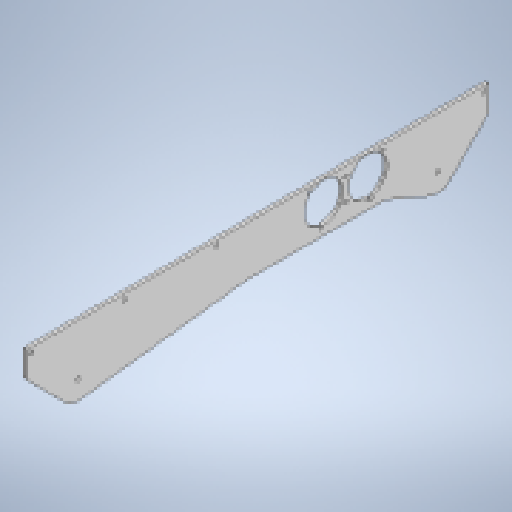
# Autodesk Inventor part: insideChassiPlate
Saved by Autodesk Inventor 2023 (Build 270158000, 158)
## iProperties
Created: 2022-09-05
Part Number: insideChassiPlate
Material: Generic
Document SubType Name: Modeling
Designer: deli
Density: 1 g/cm^3
Appearance: Default
Author: deli
Autodesk Inventor part; units mm, degrees
ref_plane "YZ Plane" through (0, 0, 0) normal (1, 0, 0) x (0, 1, 0)
ref_plane "XZ Plane" through (0, 0, 0) normal (0, 1, 0) x (-1, 0, 0)
ref_plane "XY Plane" through (0, 0, 0) normal (0, 0, 1) x (1, 0, 0)
sketch "Sketch1" plane through (0, 0, 0) normal (1, 0, 0) x (0, 1, 0)
  arc A0 (69.2168, 91.095) -> (63.9756, 76.3164) centre (81.867, 78.2899) ccw projected
  line L0 (63.9756, 76.3164) -> (81.867, -85.8871) projected
  line L1 (81.867, -85.8871) -> (81.867, -221.4489) projected
  line L2 (81.867, -221.4489) -> (65.0609, -265.2638) projected
  arc A1 (65.0609, -265.2638) -> (69.2168, -284.5152) centre (81.867, -271.7101) ccw projected
  line L3 (69.2168, -284.5152) -> (106.867, -321.7101) projected
  line L4 (106.867, -321.7101) -> (131.867, -321.7101) projected
  line L5 (131.867, -321.7101) -> (131.867, 128.2899) projected
  line L6 (131.867, 128.2899) -> (106.867, 128.2899) projected
  line L7 (106.867, 128.2899) -> (69.2168, 91.095) projected
  circle A2 centre (81.867, -271.7101) radius 2 projected
  circle A3 centre (109.117, -161.4993) radius 7 projected
  circle A4 centre (109.117, -202.8891) radius 7 projected
  circle A5 centre (81.867, 78.2899) radius 2 projected
  circle A6 centre (109.117, -161.4993) radius 19
  circle A7 centre (109.117, -202.8891) radius 19
  circle A8 centre (126.867, -217.9058) radius 2 projected
  circle A9 centre (126.867, -146.4827) radius 2 projected
  circle A10 centre (126.0665, -182.1942) radius 2 projected
  circle A11 centre (92.1676, -182.1942) radius 2 projected
  circle A12 centre (87.367, -153.2835) radius 2 projected
  circle A13 centre (87.367, -211.105) radius 2 projected
  circle A14 centre (126.867, -56.5585) radius 2 projected
  circle A15 centre (126.867, -316.7101) radius 2 projected
  circle A16 centre (126.867, 123.2899) radius 2 projected
  circle A17 centre (126.867, 33.3657) radius 2 projected
  point P0 (0, 0)
  dimension "d0" = 38
  dimension "d1" = 38
  constraints: 2 centre point, 2 coincident
  measures "d0" diameter of A6
  measures "d1" diameter of A7
extrude "Extrusion1" add sketch "Sketch1" along normal blind 3.175 contours L7 L6 L5 L4 L3 A1 L2 L1 L0 A0
equation "\"d1\" = d0"
body "Solid1"
